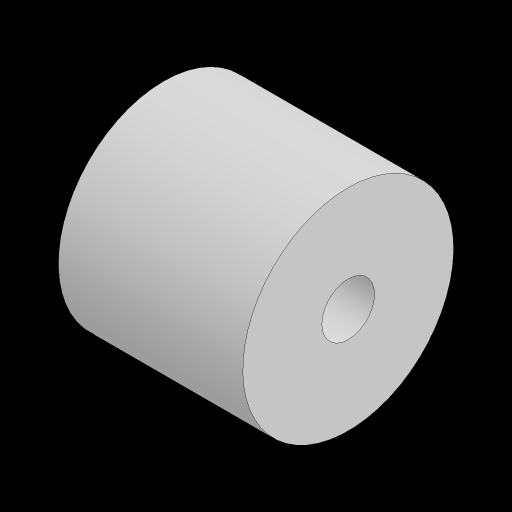
# Autodesk Inventor part: thread test
Saved by Autodesk Inventor 2023.2 (Build 272271030, 271C)
## iProperties
Created: 2023-11-11
Part Number: thread test
Material: Generic
Document SubType Name: Modeling
Designer: robpl
Density: 1 g/cm^3
Appearance: Default
Author: robpl
## iProperties of the stored document thread test_3DPrint.ipt
Created: 2023-11-11
Part Number: thread test_3DPrint
Material: Generic
Document SubType Name: Modeling
Designer: robpl
Density: 1 g/cm^3
Appearance: Default
Author: robpl
Autodesk Inventor part; units mm, degrees
ref_plane "YZ Plane" through (0, 0, 0) normal (1, 0, 0) x (0, 1, 0)
ref_plane "XZ Plane" through (0, 0, 0) normal (0, 1, 0) x (-1, 0, 0)
ref_plane "XY Plane" through (0, 0, 0) normal (0, 0, 1) x (1, 0, 0)
sketch "Sketch1" plane through (0, 0, 0) normal (0, 0, 1) x (1, 0, 0)
  line L0 (0, 0) -> (7, 0)
  line L1 (7, 0) -> (7, 4)
  line L2 (7, 4) -> (0, 4)
  line L3 (0, 4) -> (0, 0)
  line L4 (0, 0) -> (4, 0)
  line L5 (4, 0) -> (4, 2.25)
  line L6 (4, 2.25) -> (0, 2.25)
  line L7 (0, 2.25) -> (0, 0)
  line L8 (4, 0) -> (7, 0)
  line L9 (7, 0) -> (7, 1)
  line L10 (7, 1) -> (4, 1)
  line L11 (4, 1) -> (4, 0)
  dimension "d0" = 4
  dimension "d1" = 2.25
  dimension "d2" = 1
  dimension "d3" = 3
  dimension "d4" = 4
  constraints: 24 end point, 6 parallel, 3 horizontal, 3 perpendicular, 1 point on line
  measures "d0" distance of L5.end L6.end
  measures "d1" distance of L4.end L5.end
  measures "d2" distance between parallel lines of L0 L10
  measures "d3" distance of L9.end L10.end
  measures "d4" distance of L0.end L1.end
revolve "Revolution1" add sketch "Sketch1" angle 360 about axis through (0, 0, 0) along (1, 0, 0) contours L3 L2 L1 L10 L5 L6
body "Solid1"
